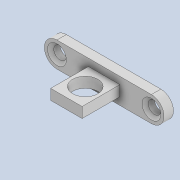
# Autodesk Inventor part: supporto asta
Saved by Autodesk Inventor 2022 (Build 260153000, 153)
## iProperties
Created: 2025-07-13
Part Number: supporto asta
Material: Generic
Document SubType Name: Modeling
Designer: 1234
Density: 1 g/cm^3
Appearance: Default
Author: 1234
Autodesk Inventor part; units mm, degrees
ref_plane "YZ Plane" through (0, 0, 0) normal (1, 0, 0) x (0, 1, 0)
ref_plane "XZ Plane" through (0, 0, 0) normal (0, 1, 0) x (-1, 0, 0)
ref_plane "XY Plane" through (0, 0, 0) normal (0, 0, 1) x (1, 0, 0)
sketch "Sketch1" plane through (0, 0, 0) normal (0, 0, 1) x (1, 0, 0)
  circle A0 centre (0, 0) radius 2
  circle A1 centre (30, 0) radius 2
  line L0 (0, 0) -> (32, 0) construction
  arc A2 (4, 0) -> (0, -4) centre (0, 0) ccw
  arc A3 (30, -4) -> (26, 0) centre (30, 0) ccw
  line L1 (30, 4) -> (0, 4)
  line L2 (0, -4) -> (30, -4)
  dimension "d1" = 4
  dimension "d0" = 4
  dimension "d2" = 30
  dimension "d3" = 8
  dimension "d4" = 8
  constraints: 6 end point, 6 point on circle, 3 centre point, 3 coincident, 3 horizontal, 3 point on line, 2 tangent, 1 horizontal alignment, 2 other
  measures "d0" diameter of A0
  measures "d2" distance of point (0, 0) point (30, 0)
  measures "d3" diameter of A2
  measures "d4" diameter of A3
extrude "Extrusion1" add sketch "Sketch1" along normal blind 3
sketch "Sketch2" plane through (0, 0, 3) normal (0, 0, 1) x (1, 0, 0)
  line L0 (10.0124, 1.7111) -> (19.9876, 1.7111)
  line L1 (19.9876, 1.7111) -> (19.9876, -1.6019)
  line L2 (19.9876, -1.6019) -> (10.0124, -1.6019)
  line L3 (10.0124, -1.6019) -> (10.0124, 1.7111)
  line L4 (15, -1.6019) -> (15, 2.8215) construction
  line L5 (0, -4) -> (30, -4) projected
  line L6 (15, -4) -> (15, 4) construction
  line L7 (30, 4) -> (0, 4) projected
  point P0 (0, 0)
  constraints: 12 end point, 3 midpoint, 2 parallel, 1 collinear, 1 horizontal, 1 perpendicular, 1 vertical
extrude "Extrusion2" add sketch "Sketch2" along normal blind 12
sketch "Sketch3" plane through (10.0124, 1.7111, 3) normal (0, 1, 0) x (1, 0, 0)
  line L0 (19.9876, 3) -> (-10.0124, 3) projected
  line L1 (4.9876, 3) -> (4.9876, -10.3246) construction
  circle A0 centre (4.9876, -6) radius 4
  dimension "d9" = 8
  dimension "d12" = 9
  constraints: 2 end point, 1 centre point, 1 midpoint, 1 point on line, 1 vertical
  measures "d9" diameter of A0
  measures "d12" distance from line of L0 A0.centre
extrude "Extrusion3" cut sketch "Sketch3" against normal blind 8
chamfer "Chamfer1" distance 1 angle 45 2 edges at (-2, 0, 3) (28, 0, 3)
body "Solid1"
